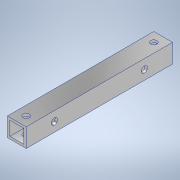
# Autodesk Inventor part: 上下直動9x9_1_CPY
Saved by Autodesk Inventor 2020.3 (Build 243373000, 373)
## iProperties
Created: 2020-07-05
Part Number: 上下直動9x9_1_CPY
Material: アルミニウム 6061
Document SubType Name: Modeling
Designer: totot
Mass: 5.97367 g
Surface Area: 38.0757 cm^2
Volume: 2.21247 cm^3
Density: 2.7 g/cm^3
Appearance: アルミニウム - フラット
Author: totot
Autodesk Inventor part; units mm, degrees
ref_plane "YZ Plane" through (0, 0, 0) normal (1, 0, 0) x (0, 1, 0)
ref_plane "XZ Plane" through (0, 0, 0) normal (0, 1, 0) x (-1, 0, 0)
ref_plane "XY Plane" through (0, 0, 0) normal (0, 0, 1) x (1, 0, 0)
sketch "スケッチ1" plane through (0, 0, 0) normal (0, 0, 1) x (1, 0, 0)
  line L0 (0, 0) -> (9, 0)
  line L1 (9, 0) -> (9, -9)
  line L2 (9, -9) -> (0, -9)
  line L3 (0, -9) -> (0, 0)
  line L4 (1.2, -1.2) -> (7.8, -1.2)
  line L5 (7.8, -1.2) -> (7.8, -7.8)
  line L6 (7.8, -7.8) -> (1.2, -7.8)
  line L7 (1.2, -7.8) -> (1.2, -1.2)
  dimension "d0" = 9
  dimension "d1" = 9
  dimension "d2" = 6.6
  dimension "d3" = 6.6
  dimension "d4" = 1.2
  dimension "d5" = 1.2
  constraints: 16 end point, 4 parallel, 2 horizontal, 2 perpendicular
  measures "d0" distance of L1.end L2.end
  measures "d1" distance of L0.end L1.end
  measures "d2" distance of L5.end L6.end
  measures "d3" distance of L4.end L5.end
  measures "d4" distance between parallel lines of L3 L7
  measures "d5" distance between parallel lines of L4 L0
extrude "押し出し1" add sketch "スケッチ1" along normal blind 70
sketch "スケッチ3" plane through (0, -9, 0) normal (0, -1, 0) x (1, 0, 0)
  line L0 (0, 70) -> (9, 70) projected
  line L1 (0, 0) -> (9, 0) projected
  line L2 (9, 0) -> (9, 70) projected
  point P0 (4.5, 4.5)
  point P1 (4.5, 65.5)
  dimension "d20" = 4.5
  dimension "d21" = 4.5
  dimension "d22" = 4.5
  dimension "d23" = 4.5
  measures "d20" distance from line of point (4.5, 65.5) L0
  measures "d21" distance from line of L1 point (4.5, 4.5)
  measures "d22" distance from line of point (4.5, 4.5) L2
  measures "d23" distance from line of point (4.5, 65.5) L2
hole "穴2" at (4.5, -9, 4.5) at (4.5, -9, 65.5) direction (0, 1, 0) diameter 3 end through all
sketch "スケッチ4" plane through (9, -9, 0) normal (1, 0, 0) x (0, 0, -1)
  line L0 (0, 0) -> (0, 9) projected
  line L1 (-70, 0) -> (-70, 9) projected
  line L2 (0, 0) -> (-70, 0) projected
  point P0 (-13.5, 4.5)
  point P1 (-56.5, 4.5)
  dimension "d31" = 13.5
  dimension "d32" = 13.5
  dimension "d33" = 4.5
  dimension "d34" = 4.5
  measures "d31" distance from line of point (-13.5, 4.5) L0
  measures "d32" distance from line of point (-56.5, 4.5) L1
  measures "d33" distance from line of L2 point (-56.5, 4.5)
  measures "d34" distance from line of L2 point (-13.5, 4.5)
hole "穴3" at (9, -4.5, 13.5) at (9, -4.5, 56.5) direction (-1, 0, 0) diameter 3 end through all
equation "\"d22\" = d21"
equation "\"d23\" = d20"
equation "\"d32\" = d31"
equation "\"d34\" = d33"
